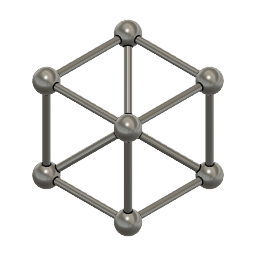
体心立方格子(40^3mm^3 スケール) (Autodesk Fusion 360 design; units mm, degrees)
Autodesk Fusion 360 part; units mm, degrees
sphere "球プリミティブ1" add diameter 10 placed x (1, 0, 0) y (0, 0, -1) z (0, 1, 0) at (0, 0, 0) makes body 1
sketch "スケッチ2" plane through (0, 0, 0) normal (0, 1, 0) x (1, 0, 0)
  line L0 (20, -20) -> (-20, -20)
  line L1 (-20, -20) -> (-20, 20)
  line L2 (-20, 20) -> (20, 20)
  line L3 (20, 20) -> (20, -20)
  line L4 (20, -20) -> (-20, 20) construction
  line L5 (-20, -20) -> (20, 20) construction
  constraint horizontal L0
  constraint perpendicular L0 L1
  constraint parallel L0 L2
  constraint parallel L1 L3
  constraint coincident L4 origin
  constraint coincident L5 origin
sketch "スケッチ3" plane through (0, 0, 0) normal (0, 0, 1) x (1, 0, 0)
extrude "押し出し1" add sketch "スケッチ2" along normal mid plane 40 separate body makes body 2
sphere "球プリミティブ2" add diameter 10 placed x (-1, 0, 0) y (0, 0, 1) z (0, 1, 0) at (20, 20, 20) separate body makes body 3
copy_body "ボディのコピーと貼り付け1" bodies 3 makes body 4
move_body "移動1" bodies 4 to x (1, 0, 0) y (0, 1, 0) z (0, 0, 1) at (0, 0, -40)
copy_body "ボディのコピーと貼り付け2" bodies 4 makes body 5
move_body "移動2" bodies 5 to x (1, 0, 0) y (0, 1, 0) z (0, 0, 1) at (-40, 0, 0)
copy_body "ボディのコピーと貼り付け3" bodies 5 makes body 6
move_body "移動3" bodies 6 to x (1, 0, 0) y (0, 1, 0) z (0, 0, 1) at (0, 0, 40)
copy_body "ボディのコピーと貼り付け4" bodies 5 6 3 4 makes body 7 makes body 8 makes body 9 makes body 10
move_body "移動4" bodies 7 8 9 10 to x (1, 0, 0) y (0, 1, 0) z (0, 0, 1) at (0, -40, 0)
sketch "スケッチ5" plane through (0, 0, 0) normal (0, 0, 1) x (1, 0, 0)
  circle A0 centre (20, 20) radius 1.5
  dimension "d5" = 3
  measures "d5" diameter of A0
extrude "押し出し2" add sketch "スケッチ5" along normal mid plane 40 separate body makes body 11
copy_body "ボディのコピーと貼り付け5" bodies 11 makes body 12
move_body "移動5" bodies 12 to x (1, 0, 0) y (0, 1, 0) z (0, 0, 1) at (-40, 0, 0)
copy_body "ボディのコピーと貼り付け6" bodies 12 11 makes body 13 makes body 14
move_body "移動6" bodies 13 14 to x (1, 0, 0) y (0, 1, 0) z (0, 0, 1) at (0, -40, 0)
copy_body "ボディのコピーと貼り付け7" bodies 11 12 14 13 makes body 15 makes body 16 makes body 17 makes body 18
move_body "移動7" bodies 15 16 17 18 to x (0, 0, 1) y (0, 1, 0) z (-1, 0, 0) at (0, 0, 0)
copy_body "ボディのコピーと貼り付け8" bodies 11 16 15 12 makes body 19 makes body 20 makes body 21 makes body 22
move_body "移動8" bodies 19 20 21 22 to x (0, 1, 0) y (-1, 0, 0) z (0, 0, 1) at (40, 0, 0)
copy_body "ボディのコピーと貼り付け9" bodies 16 11 15 12 makes body 23 makes body 24 makes body 25 makes body 26
move_body "移動9" bodies 23 24 25 26 to x (1, 0, 0) y (0, 0, 1) z (0, -1, 0) at (0, 0, -40)
copy_body "ボディのコピーと貼り付け10" bodies 21 makes body 27
move_body "移動10" bodies 27 to x (1, 0, 0) y (0, 1, 0) z (0, 0, 1) at (-40, 0, 0)
sketch "スケッチ6" plane through (0, 0, 0) normal (0, 0, 1) x (1, 0, 0)
  circle A0 centre (-20, -20) radius 1.5
  dimension "d11" = 3
  measures "d11" diameter of A0
extrude "押し出し3" add sketch "スケッチ6" along normal blind 20 and the other way blind 50 separate body makes body 28
move_body "移動11" bodies 28 to x (0.707107, 0, 0.707107) y (-0.408248, 0.816496, 0.408248) z (-0.57735, -0.577351, 0.57735) at (-2.4758, 7.8769, 30.7601)
combine "結合1" operation add target body 28 tool bodies 1
copy_body "ボディのコピーと貼り付け11" bodies 28 makes body 29
move_body "移動12" bodies 29 to x (0, 0, 1) y (0, 1, 0) z (-1, 0, 0) at (0, 0, 0)
copy_body "ボディのコピーと貼り付け12" bodies 28 29 makes body 30 makes body 31
move_body "移動13" bodies 30 31 to x (-1, 0, 0) y (0, 1, 0) z (0, 0, -1) at (0, 0, 0)
combine "結合2" operation add target body 3 tool bodies 4 13 18 6 19 15 23 22 14 21 12 20 7 5 11 17 9 24 25 26 27 29 10 31 28 30 8 16
hidden bodies 2
named bodies: "体心立方格子"
